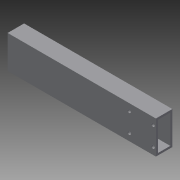
# Autodesk Inventor part: Modified Front Frame 27 in
Saved by Autodesk Inventor 2015 (Build 190159000, 159)
## iProperties
Created: 2015-01-21
Part Number: Modified Front Frame 27 in
Material: Generic
Document SubType Name: Modeling
Designer: chapale16
Density: 1 g/cm^3
Appearance: Default
Author: chapale16
Autodesk Inventor part; units mm, degrees
ref_plane "YZ Plane" through (0, 0, 0) normal (1, 0, 0) x (0, 1, 0)
ref_plane "XZ Plane" through (0, 0, 0) normal (0, 1, 0) x (-1, 0, 0)
ref_plane "XY Plane" through (0, 0, 0) normal (0, 0, 1) x (1, 0, 0)
sketch "Sketch1" plane through (0, 0, 0) normal (1, 0, 0) x (0, 1, 0)
  line L0 (0, 0) -> (50.8, 0)
  line L1 (50.8, 0) -> (50.8, -25.4)
  line L2 (50.8, -25.4) -> (0, -25.4)
  line L3 (0, -25.4) -> (0, 0)
  line L4 (47.625, -22.225) -> (47.625, -3.175)
  line L5 (47.625, -3.175) -> (3.175, -3.175)
  line L6 (3.175, -3.175) -> (3.175, -22.225)
  line L7 (3.175, -22.225) -> (47.625, -22.225)
  dimension "d0" = 50.8
  dimension "d1" = 25.4
  dimension "d2" = 3.175
  constraints: 16 end point, 4 parallel, 2 perpendicular, 1 horizontal, 3 other
  measures "d0" distance of L1.end L2.end
  measures "d1" distance of L0.end L1.end
  measures "d2" distance between parallel lines of L1 L4
extrude "Extrusion1" add sketch "Sketch1" along normal blind 685.8
sketch "Sketch2" plane through (0, 50.8, 0) normal (0, 1, 0) x (1, 0, 0)
  line L0 (0, 0) -> (0, 25.4) projected
  line L1 (0, 0) -> (685.8, 0) projected
  line L2 (685.8, 25.4) -> (685.8, 0) projected
  line L3 (0, 25.4) -> (685.8, 25.4) projected
  line L4 (0, 0) -> (685.8, 0) projected
  line L5 (228.6, 0) -> (685.8, 0)
  line L6 (685.8, 0) -> (685.8, 25.4)
  line L7 (685.8, 25.4) -> (228.6, 25.4)
  line L8 (228.6, 25.4) -> (228.6, 0)
  constraints: 8 end point, 2 parallel, 1 horizontal, 1 perpendicular, 1 point on line
extrude "Extrusion2" cut sketch "Sketch2" against normal blind 685.8 contours L8 L3 L2 L1
hole "Hole1" at (224.155, 40.005, 0) direction (0, 0, -1) diameter 5.08 depth 12.7 tip angle 118
hole "Hole2" at (224.155, 10.795, 0) direction (0, 0, -1) diameter 5.08 depth 12.7 tip angle 118
pattern_linear "Rectangular Pattern1" count 2 spacing 36.83 along (-1, 0, 0) of "Hole1"
pattern_linear "Rectangular Pattern2" count 2 spacing 36.83 along (-1, 0, 0) of "Hole2"
body "Solid1"
